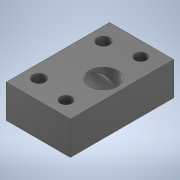
# Autodesk Inventor part: Feeder2
Saved by Autodesk Inventor 2020.2 (Build 242310000, 310)
## iProperties
Created: 2020-10-21
Part Number: Feeder2
Material: Generic
Document SubType Name: Modeling
Designer: JK
Density: 1 g/cm^3
Appearance: Smooth - Black
Author: JK
Autodesk Inventor part; units mm, degrees
ref_plane "YZ Plane" through (0, 0, 0) normal (1, 0, 0) x (0, 1, 0)
ref_plane "XZ Plane" through (0, 0, 0) normal (0, 1, 0) x (-1, 0, 0)
ref_plane "XY Plane" through (0, 0, 0) normal (0, 0, 1) x (1, 0, 0)
sketch "Sketch1" plane through (0, 0, 0) normal (0, 1, 0) x (-1, 0, 0)
  circle A0 centre (0, 0) radius 6.75
  circle A1 centre (0, 18) radius 2.75
  circle A2 centre (15.5, 15.5) radius 1.85
  circle A3 centre (15.5, -15.5) radius 1.85
  circle A4 centre (0, -18) radius 2.75
  line L0 (21.85, 24.85) -> (-9, 24.85)
  line L1 (-9, 24.85) -> (-9, -24.85)
  line L2 (-9, -24.85) -> (21.85, -24.85)
  line L3 (21.85, -24.85) -> (21.85, 24.85)
  dimension "d0" = 13.5
  dimension "d1" = 18
  dimension "d2" = 5.5
  dimension "d3" = 18
  dimension "d4" = 31
  dimension "d5" = 3.7
  dimension "d6" = 15.5
  dimension "d7" = 15.5
  dimension "d8" = 9
  dimension "d9" = 49.7
  dimension "d10" = 24.85
  dimension "d11" = 21.85
  constraints: 8 end point, 5 centre point, 2 equal radius, 2 parallel, 1 coincident, 1 horizontal, 1 perpendicular, 1 vertical alignment
  measures "d0" diameter of A0
  measures "d1" distance of point (0, 0) A1.centre
  measures "d2" diameter of A1
  measures "d3" distance of point (0, 0) A4.centre
  measures "d4" distance of A3.centre A2.centre
  measures "d5" diameter of A2
  measures "d6" horizontal distance of A2.centre point (0, 0)
  measures "d7" horizontal distance of A3.centre point (0, 0)
  measures "d8" distance from line of point (0, 0) L1
  measures "d9" distance between parallel lines of L2 L0
  measures "d10" distance from line of L2 point (0, 0)
  measures "d11" distance from line of point (0, 0) L3
extrude "Extrusion1" add sketch "Sketch1" along normal blind 16
sketch "Sketch2" plane through (-21.85, 0, -24.85) normal (-1, 0, 0) x (0, 0, 1)
  circle A0 centre (24.85, 8) radius 6.75
  point P0 (24.85, 0)
  dimension "d14" = 13.5
  dimension "d15" = 8
  constraints: 1 centre point
  measures "d14" diameter of A0
  measures "d15" distance of point (24.85, 0) A0.centre
extrude "Extrusion2" cut sketch "Sketch2" against normal blind 21.85
sketch "Sketch3" plane through (0, 0, 0) normal (0, -1, 0) x (1, 0, 0)
  circle A0 centre (0, -18) radius 2.75 projected
  circle A1 centre (0, -18) radius 4.55
  circle A2 centre (0, 18) radius 2.75 projected
  circle A3 centre (0, 18) radius 4.55
  line L0 (-4.55, -18) -> (-2.275, -14.0596)
  line L1 (-2.275, -14.0596) -> (2.275, -14.0596)
  line L2 (2.275, -14.0596) -> (4.55, -18)
  line L3 (4.55, -18) -> (2.275, -21.9404)
  line L4 (2.275, -21.9404) -> (-2.275, -21.9404)
  line L5 (-2.275, -21.9404) -> (-4.55, -18)
  line L6 (-4.55, 18) -> (-2.275, 21.9404)
  line L7 (-2.275, 21.9404) -> (2.275, 21.9404)
  line L8 (2.275, 21.9404) -> (4.55, 18)
  line L9 (4.55, 18) -> (2.275, 14.0596)
  line L10 (2.275, 14.0596) -> (-2.275, 14.0596)
  line L11 (-2.275, 14.0596) -> (-4.55, 18)
  point P0 (0, 0)
  dimension "d18" = 9.1
  constraints: 24 end point, 4 coincident, 4 horizontal alignment, 30 other
extrude "Extrusion3" cut sketch "Sketch3" against normal blind 4 contours L3 L4 L5 L0 L1 L2 | L9 L10 L11 L6 L7 L8
sketch "Sketch4" plane through (0, 16, 0) normal (0, 1, 0) x (1, 0, 0)
  circle A0 centre (-15.5, -15.5) radius 1.85 projected
  circle A1 centre (-15.5, -15.5) radius 3
  circle A2 centre (-15.5, 15.5) radius 1.85 projected
  circle A3 centre (-15.5, 15.5) radius 3
  point P0 (0, 0)
  dimension "d21" = 6
  constraints: 2 centre point, 2 coincident, 1 equal radius
  measures "d21" diameter of A1
extrude "Extrusion4" cut sketch "Sketch4" against normal blind 4 contours A0 | A1 | A2 | A3
body "Solid1"
